Mount_Fit_Test (Autodesk Fusion 360 design; units mm, degrees)
part number: 2026-09-18-15-11-56-161
Autodesk Fusion 360 part; units mm, degrees
sketch "Sketch1" plane through (0, 0, 0) normal (0, 0, 1) x (1, 0, 0)
  line L0 (0, 0) -> (125, 0)
  line L1 (125, 0) -> (125, -75)
  line L2 (125, -75) -> (0, -75)
  line L3 (0, -75) -> (0, 0)
  constraint horizontal L0
  constraint vertical L1
  constraint horizontal L2
  constraint vertical L3
  constraint coincident L0.start L3.end
extrude "Extrude1" add sketch "Sketch1" along normal blind 5
extrude "Extrude2" cut 1 faces at (125, -25, 3.3333) along direction (-1, 0, 0) blind 44
